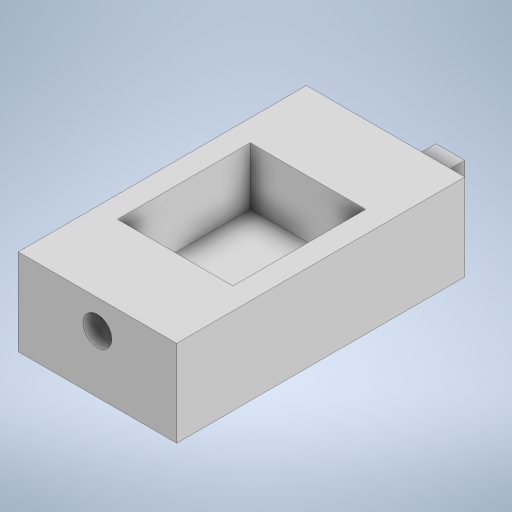
# Autodesk Inventor part: camera_support_2
Saved by Autodesk Inventor 2023 (Build 270158000, 158)
## iProperties
Created: 2022-07-04
Part Number: camera_support_2
Material: Genérico
Document SubType Name: Modeling
Designer: inigo
Density: 1 g/cm^3
Appearance: Valor por defecto
Author: inigo
Autodesk Inventor part; units mm, degrees
ref_plane "YZ Plane" through (0, 0, 0) normal (1, 0, 0) x (0, 1, 0)
ref_plane "XZ Plane" through (0, 0, 0) normal (0, 1, 0) x (-1, 0, 0)
ref_plane "XY Plane" through (0, 0, 0) normal (0, 0, 1) x (1, 0, 0)
sketch "Boceto1" plane through (0, 0, 0) normal (0, 1, 0) x (-1, 0, 0)
  line L0 (27.5, 50) -> (-27.5, 50)
  line L1 (-27.5, 50) -> (-27.5, -50)
  line L2 (-27.5, -50) -> (27.5, -50)
  line L3 (27.5, -50) -> (27.5, 50)
  line L4 (27.5, 50) -> (-27.5, -50) construction
  line L5 (-27.5, 50) -> (27.5, -50) construction
  point P0 (0, 0)
  dimension "d0" = 55
  dimension "d1" = 100
  constraints: 12 end point, 2 midpoint, 2 parallel, 1 horizontal, 1 perpendicular
  measures "d0" distance of L2.end L1.end
  measures "d1" distance of L1.end L0.end
extrude "Extrusión1" add sketch "Boceto1" along normal blind 30
sketch "Boceto2" plane through (27.5, 0, -50) normal (0, 0, -1) x (-1, 0, 0)
  line L0 (10, 25) -> (20, 25)
  line L1 (20, 25) -> (20, 15)
  line L2 (20, 15) -> (10, 15)
  line L3 (10, 15) -> (10, 25)
  line L4 (10, 25) -> (20, 15) construction
  line L5 (20, 25) -> (10, 15) construction
  line L6 (0, 30) -> (55, 30) projected
  line L7 (0, 0) -> (0, 30) projected
  point P0 (27.5, 0)
  point P1 (15, 20)
  point P2 (15, 25)
  dimension "d4" = 10
  dimension "d5" = 10
  dimension "d6" = 5
  dimension "d7" = 10
  constraints: 12 end point, 3 midpoint, 2 parallel, 1 horizontal, 1 perpendicular
  measures "d4" distance of L1.end L2.end
  measures "d5" distance of L0.end L1.end
  measures "d6" distance from line of L6 point (15, 25)
  measures "d7" distance between parallel lines of L3 L7
extrude "Extrusión2" add sketch "Boceto2" along normal blind 10
sketch "Boceto3" plane through (-27.5, 0, 50) normal (0, 0, 1) x (1, 0, 0)
  circle A0 centre (27.5, 20) radius 5
  line L0 (0, 30) -> (55, 30) projected
  point P0 (27.5, 0)
  point P1 (27.5, 30)
  dimension "d10" = 10
  dimension "d11" = 10
  constraints: 1 centre point, 1 midpoint
  measures "d10" diameter of A0
  measures "d11" distance of point (27.5, 30) A0.centre
extrude "Extrusión3" cut sketch "Boceto3" against normal blind 15
sketch "Boceto4" plane through (0, 30, 0) normal (0, 1, 0) x (1, 0, 0)
  line L0 (-20, 23) -> (20, 23)
  line L1 (20, 23) -> (20, -23)
  line L2 (20, -23) -> (-20, -23)
  line L3 (-20, -23) -> (-20, 23)
  line L4 (-20, 23) -> (20, -23) construction
  line L5 (20, 23) -> (-20, -23) construction
  point P0 (0, 0)
  dimension "d14" = 40
  dimension "d15" = 46
  constraints: 12 end point, 2 midpoint, 2 parallel, 1 horizontal, 1 perpendicular
  measures "d14" distance of L1.end L2.end
  measures "d15" distance of L0.end L1.end
extrude "Extrusión4" cut sketch "Boceto4" against normal blind 20
